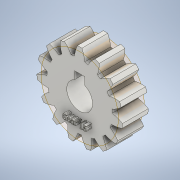
# Autodesk Inventor part: Spur Gear15
Saved by Autodesk Inventor 2021 (Build 250183000, 183)
## iProperties
CustomPartVersion: 1
Created: 2021-04-10
Part Number: Spur Gear15
Material: Steel
Document SubType Name: Modeling
Designer: Nabeel Azafer
Categories: <?xml version="1.0" encoding="UTF-16"?> <MemberInstance><Categories><FamilyTemplate><FamilyTemplateParameter ValueType="xs:double" Id="1" ObjectReferenceKey="da_z" ObjectType="kUserParameterObject"/><FamilyTemplateParameter ValueType="xs:double" Id="2" ObjectReferenceKey="da_b" ObjectType="kUserParameterObject"/><FamilyTemplateParameter ValueType="xs:double" Id="3" ObjectReferenceKey="da_beta" ObjectType="kUserParameterObject"/><FamilyTemplateParameter ValueType="xs:double" Id="4" ObjectReferenceKey="da_da" ObjectType="kUserParameterObject"/><FamilyTemplateParameter ValueType="xs:double" Id="5" ObjectReferenceKey="da_aw" ObjectType="kUserParameterObject"/><FamilyTemplateParameter ValueType="xs:string" Id="6" ObjectReferenceKey="EAIAABAAAACIAQAAAAAAAIAAAAAAAAAA" ObjectType="83910656" SubObjectId="SurfaceGeometry"/></FamilyTemplate><ParamToTemplateMap><ParamToTemplate CategoryParameter="//CategoryParameter[@InternalName='046C89C9-8512-4d59-83FE-43B91F4F132A']" TemplateParameter="1"/><ParamToTemplate CategoryParameter="//CategoryParameter[@InternalName='2552DF32-E462-4b46-AEBF-C6C7768E72AC']" TemplateParameter="2"/><ParamToTemplate CategoryParameter="//CategoryParameter[@InternalName='C9EE641D-15FC-4fae-A226-E94C4372FDD7']" TemplateParameter="3"/><ParamToTemplate><ParamToTemplate CategoryParameter="//CategoryParameter[@InternalName='00B6519A-459B-49c7-AD84-2E56D39A5744']" ConstantValue="0.000000"/></ParamToTemplate><ParamToTemplate><ParamToTemplate CategoryParameter="//CategoryParameter[@InternalName='04B31F0E-C7A6-4894-AA32-9629BEFACF47']" ConstantValue="0.800000"/></ParamToTemplate><ParamToTemplate><ParamToTemplate CategoryParameter="//CategoryParameter[@InternalName='43CBEC2E-7847-49e7-A936-2F7889FCB2D9']" ConstantValue="0.350000"/></ParamToTemplate><ParamToTemplate><ParamToTemplate CategoryParameter="//CategoryParameter[@InternalName='B1EFC894-105D-4ebd-86BF-FA20ED196853']" ConstantValue="0.500000"/></ParamToTemplate><ParamToTemplate><ParamToTemplate CategoryParameter="//CategoryParameter[@InternalName='51175063-3D10-4879-93E8-6246FE8B403D']" ConstantValue="2060000000.000000"/></ParamToTemplate><ParamToTemplate><ParamToTemplate CategoryParameter="//CategoryParameter[@InternalName='A3A52E27-4454-46a9-B0BD-C932399B70AF']" ConstantValue="0.300000"/></ParamToTemplate><ParamToTemplate><ParamToTemplate CategoryParameter="//CategoryParameter[@InternalName='91B76062-C214-41d9-B1B9-14D2AB99603D']" ConstantValue="0.100000"/></ParamToTemplate><ParamToTemplate><ParamToTemplate CategoryParameter="//CategoryParameter[@InternalName='374E806E-8B8A-4dda-A9AA-1039D6500AD2']" ConstantValue="10.000000"/></ParamToTemplate><ParamToTemplate><ParamToTemplate CategoryParameter="//CategoryParameter[@InternalName='2D373A89-B862-43d6-8D0B-0CBF12AB9F6C']" ConstantValue="0.349066"/></ParamToTemplate><ParamToTemplate CategoryParameter="//CategoryParameter[@InternalName='37777632-D6A2-4fac-9D53-DB8ACD95C989']" TemplateParameter="4"/><ParamToTemplate CategoryParameter="//CategoryParameter[@InternalName='FD1017F1-B727-4f7e-9707-0F86F1FF9423']" TemplateParameter="5"/><ParamToTemplate><ParamToTemplate CategoryParameter="//CategoryParameter[@InternalName='9E1B4470-B2D3-4ff1-B813-535BB4CDF51A']" ConstantValue="3520000.000000"/></ParamToTemplate><ParamToTemplate><ParamToTemplate CategoryParameter="//CategoryParameter[@InternalName='F8452263-BFF6-458c-9FB1-07C4B99E95CD']" ConstantValue="11400000.000000"/></ParamToTemplate><ParamToTemplate><ParamToTemplate CategoryParameter="//CategoryParameter[@InternalName='3E3BB259-FD49-497f-8171-6EBC954A3479']" ConstantValue="2.000000"/></ParamToTemplate><ParamToTemplate CategoryParameter="//CategoryParameter[@InternalName='27C3BAF2-7550-4e4b-AE2C-0DB134B7D9B7']" TemplateParameter="6"/></ParamToTemplateMap><Category DisplayName="Gear" InternalName="DC85795E-93AB-48d5-8EEE-5A27447B64BD" Mnemonic="Gear"><CategoryParameter DisplayName="z" InternalName="046C89C9-8512-4d59-83FE-43B91F4F132A" Mnemonic="z"/><CategoryParameter DisplayName="b" InternalName="2552DF32-E462-4b46-AEBF-C6C7768E72AC" Mnemonic="b"/><CategoryParameter DisplayName="||b|" InternalName="C9EE641D-15FC-4fae-A226-E94C4372FDD7" Mnemonic="beta"/><CategoryParameter DisplayName="x" InternalName="00B6519A-459B-49c7-AD84-2E56D39A5744" Mnemonic="x"/><CategoryParameter DisplayName="a*" InternalName="04B31F0E-C7A6-4894-AA32-9629BEFACF47" Mnemonic="a"/><CategoryParameter DisplayName="c*" InternalName="43CBEC2E-7847-49e7-A936-2F7889FCB2D9" Mnemonic="c"/><CategoryParameter DisplayName="r|.f|*" InternalName="B1EFC894-105D-4ebd-86BF-FA20ED196853" Mnemonic="rf"/><CategoryParameter DisplayName="E" InternalName="51175063-3D10-4879-93E8-6246FE8B403D" Mnemonic="E"/><CategoryParameter DisplayName="||m|" InternalName="A3A52E27-4454-46a9-B0BD-C932399B70AF" Mnemonic="mi"/><Category DisplayName="SpurGear" InternalName="26C5A22E-A91E-4dfd-A3B3-23CCAFAE1764" Mnemonic="SpurGear"><CategoryParameter DisplayName="m" InternalName="91B76062-C214-41d9-B1B9-14D2AB99603D" Mnemonic="m"/><CategoryParameter DisplayName="P" InternalName="374E806E-8B8A-4dda-A9AA-1039D6500AD2" Mnemonic="PP"/><CategoryParameter DisplayName="||a|" InternalName="2D373A89-B862-43d6-8D0B-0CBF12AB9F6C" Mnemonic="alpha"/><CategoryParameter DisplayName="d|.a|" InternalName="37777632-D6A2-4fac-9D53-DB8ACD95C989" Mnemonic="da"/><CategoryParameter DisplayName="a|.w|" InternalName="FD1017F1-B727-4f7e-9707-0F86F1FF9423" Mnemonic="aw"/><CategoryParameter DisplayName="||s||.Flim|" InternalName="9E1B4470-B2D3-4ff1-B813-535BB4CDF51A" Mnemonic="sFlim"/><CategoryParameter DisplayName="||s||.Hlim|" InternalName="F8452263-BFF6-458c-9FB1-07C4B99E95CD" Mnemonic="sHlim"/><CategoryParameter DisplayName="type" InternalName="3E3BB259-FD49-497f-8171-6EBC954A3479" Mnemonic="type"/><CategoryParameter DisplayName="PitchDiameter" InternalName="27C3BAF2-7550-4e4b-AE2C-0DB134B7D9B7" Mnemonic="IDS_PITCHDIAM"/></Category></Category></Categories></MemberInstance>
Density: 7.85 g/cm^3
Appearance: Steel
Mass: 10.3734 g
Surface Area: 10.947 cm^2
Volume: 1.32145 cm^3
Author: Nabeel Azafer
Autodesk Inventor part; units mm, degrees
ref_plane "YZ Plane" through (0, 0, 0) normal (1, 0, 0) x (0, 1, 0)
ref_plane "XZ Plane" through (0, 0, 0) normal (0, 1, 0) x (-1, 0, 0)
ref_plane "XY Plane" through (0, 0, 0) normal (0, 0, 1) x (1, 0, 0)
sketch "Sketch1" plane through (0, 0, 0) normal (0, 0, 1) x (1, 0, 0)
  circle A0 centre (0, 0) radius 8.3
  dimension "d0" = 16.6
  constraints: 1 centre point
  measures "d0" diameter of A0
extrude "Extrusion1" add sketch "Sketch1" along normal blind 5
ref_plane "Work Plane2" through (0, 0, 2.5) normal (0, 0, 1) x (1, 0, 0)
sketch "Sketch2" plane through (0, 0, 0) normal (0, 0, -1) x (-1, 0, 0)
  circle A0 centre (0, 0) radius 8.3 projected
  circle A1 centre (0, 0) radius 7.5
  dimension "d3" = 15
  constraints: 1 centre point, 1 coincident
  measures "d3" diameter of A1
surface extrude "Pitch Diameter" sketch "Sketch2" against normal through all shown yes curves A1
ref_plane "Work Plane8" through (0, 0, 0) normal (0.9781476, 0.2079117, 0) x (0, 0, 1)
ref_plane "Work Plane9" through (0, 0, 0) normal (1, 0, 0) x (0, 1, 0)
spur gear teeth "Spur Gear" teeth 15 pitch diameter 15 tip diameter 16.6 root diameter 12.7 face width 8 start plane through (0, 0, 0) normal (0, 0, -1) x (-1, 0, 0)
sketch "Sketch4" plane through (0, 0, 5) normal (0, 0, 1) x (1, 0, 0)
  circle A0 centre (0, 0) radius 2.5
  line L0 (-1, 2.2913) -> (1, 2.2913)
  line L1 (1, 2.2913) -> (1, 3.7913)
  line L2 (1, 3.7913) -> (-1, 3.7913)
  line L3 (-1, 3.7913) -> (-1, 2.2913)
  dimension "d57" = 5
  dimension "d58" = 2
  dimension "d59" = 1.5
  constraints: 8 end point, 2 parallel, 1 coincident, 1 horizontal, 1 perpendicular, 3 other
  measures "d58" distance of L2.end L1.end
  measures "d59" distance of L1.end L0.end
extrude "Extrusion2" cut sketch "Sketch4" against normal blind 5
sketch "Sketch5" plane through (0, 0, 5) normal (0, 0, 1) x (1, 0, 0)
  line L0 (-2.4127, -3.3956) -> (4.2445, -3.3956) construction
  line L1 (4.2445, -3.3956) -> (4.2445, -5.5849) construction
  line L2 (4.2445, -5.5849) -> (-2.4127, -5.5849) construction
  line L3 (-2.4127, -5.5849) -> (-2.4127, -3.3956) construction
  spline S0 degree 2 poles (-1.8924, -4.4329) (-1.9986, -4.4329) (-2.1744, -4.3681) (-2.2376, -4.3024) knots 0 0 0 1 2 2 2
  spline S1 degree 2 poles (-2.2376, -4.3024) (-2.3008, -4.236) (-2.3681, -4.0399) (-2.3681, -3.9126) knots 0 0 0 1 2 2 2
  spline S2 degree 2 poles (-2.3681, -3.9126) (-2.3681, -3.7919) (-2.3, -3.6006) (-2.2368, -3.5326) knots 0 0 0 1 2 2 2
  spline S3 degree 2 poles (-2.2368, -3.5326) (-2.176, -3.4669) (-1.9978, -3.3956) (-1.8916, -3.3956) knots 0 0 0 1 2 2 2
  spline S4 degree 2 poles (-1.8916, -3.3956) (-1.8405, -3.3956) (-1.7482, -3.4102) (-1.706, -3.4232) knots 0 0 0 1 2 2 2
  spline S5 degree 2 poles (-1.706, -3.4232) (-1.672, -3.4329) (-1.5893, -3.4685) (-1.5642, -3.4815) knots 0 0 0 1 2 2 2
  line L4 (-1.5642, -3.4815) -> (-1.5642, -3.642)
  line L5 (-1.5642, -3.642) -> (-1.5756, -3.642)
  spline S6 degree 2 poles (-1.5756, -3.642) (-1.6007, -3.6201) (-1.6534, -3.5804) (-1.702, -3.5577) knots 0 0 0 1 2 2 2
  spline S7 degree 2 poles (-1.702, -3.5577) (-1.7425, -3.5374) (-1.847, -3.5107) (-1.907, -3.5107) knots 0 0 0 1 2 2 2
  spline S8 degree 2 poles (-1.907, -3.5107) (-2.0512, -3.5107) (-2.2295, -3.7279) (-2.2295, -3.9086) knots 0 0 0 1 2 2 2
  spline S9 degree 2 poles (-2.2295, -3.9086) (-2.2295, -4.0091) (-2.1825, -4.1598) (-2.138, -4.2117) knots 0 0 0 1 2 2 2
  spline S10 degree 2 poles (-2.138, -4.2117) (-2.095, -4.2635) (-1.9735, -4.3178) (-1.8973, -4.3178) knots 0 0 0 1 2 2 2
  spline S11 degree 2 poles (-1.8973, -4.3178) (-1.8414, -4.3178) (-1.7295, -4.3016) (-1.6914, -4.2854) knots 0 0 0 1 2 2 2
  line L6 (-1.6914, -4.2854) -> (-1.6914, -4.0269)
  line L7 (-1.6914, -4.0269) -> (-1.9232, -4.0269)
  line L8 (-1.9232, -4.0269) -> (-1.9232, -3.9102)
  line L9 (-1.9232, -3.9102) -> (-1.5602, -3.9102)
  line L10 (-1.5602, -3.9102) -> (-1.5602, -4.347)
  spline S12 degree 2 poles (-1.5602, -4.347) (-1.5853, -4.3583) (-1.6712, -4.3932) (-1.7076, -4.4037) knots 0 0 0 1 2 2 2
  spline S13 degree 2 poles (-1.7076, -4.4037) (-1.7571, -4.4183) (-1.8365, -4.4329) (-1.8924, -4.4329) knots 0 0 0 1 2 2 2
  spline S14 degree 2 poles (-1.0772, -4.4305) (-1.2571, -4.4305) (-1.4548, -4.2287) (-1.4548, -4.0423) knots 0 0 0 1 2 2 2
  spline S15 degree 2 poles (-1.4548, -4.0423) (-1.4548, -3.8591) (-1.2628, -3.642) (-1.108, -3.642) knots 0 0 0 1 2 2 2
  spline S16 degree 2 poles (-1.108, -3.642) (-1.0383, -3.642) (-0.9305, -3.6825) (-0.8908, -3.7254) knots 0 0 0 1 2 2 2
  spline S17 degree 2 poles (-0.8908, -3.7254) (-0.8503, -3.7684) (-0.8073, -3.8924) (-0.8073, -3.9823) knots 0 0 0 1 2 2 2
  line L11 (-0.8073, -3.9823) -> (-0.8073, -4.0512)
  line L12 (-0.8073, -4.0512) -> (-1.3268, -4.0512)
  spline S18 degree 2 poles (-1.3268, -4.0512) (-1.3268, -4.1817) (-1.1955, -4.3202) (-1.0788, -4.3202) knots 0 0 0 1 2 2 2
  spline S19 degree 2 poles (-1.0788, -4.3202) (-1.0375, -4.3202) (-0.9572, -4.3016) (-0.9248, -4.287) knots 0 0 0 1 2 2 2
  spline S20 degree 2 poles (-0.9248, -4.287) (-0.8908, -4.2708) (-0.8438, -4.2425) (-0.8284, -4.2295) knots 0 0 0 1 2 2 2
  line L13 (-0.8284, -4.2295) -> (-0.8211, -4.2295)
  line L14 (-0.8211, -4.2295) -> (-0.8211, -4.3673)
  spline S21 degree 2 poles (-0.8211, -4.3673) (-0.843, -4.3762) (-0.9094, -4.4021) (-0.9354, -4.4094) knots 0 0 0 1 2 2 2
  spline S22 degree 2 poles (-0.9354, -4.4094) (-0.9718, -4.4199) (-1.0318, -4.4305) (-1.0772, -4.4305) knots 0 0 0 1 2 2 2
  spline S23 degree 2 poles (-0.9305, -3.9548) (-0.9321, -3.9037) (-0.9532, -3.8292) (-0.9735, -3.804) knots 0 0 0 1 2 2 2
  spline S24 degree 2 poles (-0.9735, -3.804) (-0.9953, -3.7757) (-1.0642, -3.7457) (-1.1153, -3.7457) knots 0 0 0 1 2 2 2
  spline S25 degree 2 poles (-1.1153, -3.7457) (-1.1655, -3.7457) (-1.236, -3.7757) (-1.2652, -3.8049) knots 0 0 0 1 2 2 2
  spline S26 degree 2 poles (-1.2652, -3.8049) (-1.2935, -3.8348) (-1.3227, -3.907) (-1.3268, -3.9548) knots 0 0 0 1 2 2 2
  line L15 (-1.3268, -3.9548) -> (-0.9305, -3.9548)
  spline S27 degree 2 poles (-0.2611, -4.334) (-0.2765, -4.3454) (-0.3284, -4.3859) (-0.3527, -4.398) knots 0 0 0 1 2 2 2
  spline S28 degree 2 poles (-0.3527, -4.398) (-0.3859, -4.4159) (-0.4483, -4.4345) (-0.5051, -4.4345) knots 0 0 0 1 2 2 2
  spline S29 degree 2 poles (-0.5051, -4.4345) (-0.5512, -4.4345) (-0.6347, -4.3997) (-0.6663, -4.3681) knots 0 0 0 1 2 2 2
  spline S30 degree 2 poles (-0.6663, -4.3681) (-0.6963, -4.3373) (-0.7328, -4.2465) (-0.7328, -4.1963) knots 0 0 0 1 2 2 2
  spline S31 degree 2 poles (-0.7328, -4.1963) (-0.7328, -4.1185) (-0.6671, -4.0083) (-0.5958, -3.9767) knots 0 0 0 1 2 2 2
  spline S32 degree 2 poles (-0.5958, -3.9767) (-0.5326, -3.9475) (-0.3608, -3.9256) (-0.2611, -3.9199) knots 0 0 0 1 2 2 2
  line L16 (-0.2611, -3.9199) -> (-0.2611, -3.8956)
  spline S33 degree 2 poles (-0.2611, -3.8956) (-0.2611, -3.8519) (-0.2879, -3.7976) (-0.3122, -3.7822) knots 0 0 0 1 2 2 2
  spline S34 degree 2 poles (-0.3122, -3.7822) (-0.3365, -3.7668) (-0.4062, -3.757) (-0.4435, -3.757) knots 0 0 0 1 2 2 2
  spline S35 degree 2 poles (-0.4435, -3.757) (-0.4872, -3.757) (-0.6055, -3.783) (-0.6647, -3.8081) knots 0 0 0 1 2 2 2
  line L17 (-0.6647, -3.8081) -> (-0.672, -3.8081)
  line L18 (-0.672, -3.8081) -> (-0.672, -3.6792)
  spline S36 degree 2 poles (-0.672, -3.6792) (-0.6371, -3.6695) (-0.5067, -3.6452) (-0.4427, -3.6452) knots 0 0 0 1 2 2 2
  spline S37 degree 2 poles (-0.4427, -3.6452) (-0.3649, -3.6452) (-0.2587, -3.6695) (-0.2166, -3.7011) knots 0 0 0 1 2 2 2
  spline S38 degree 2 poles (-0.2166, -3.7011) (-0.1752, -3.7319) (-0.1347, -3.83) (-0.1347, -3.9005) knots 0 0 0 1 2 2 2
  line L19 (-0.1347, -3.9005) -> (-0.1347, -4.4134)
  line L20 (-0.1347, -4.4134) -> (-0.2611, -4.4134)
  line L21 (-0.2611, -4.4134) -> (-0.2611, -4.334)
  line L22 (-0.2611, -4.2287) -> (-0.2611, -4.0204)
  spline S39 degree 2 poles (-0.2611, -4.0204) (-0.3065, -4.0245) (-0.4435, -4.0382) (-0.4864, -4.0512) knots 0 0 0 1 2 2 2
  spline S40 degree 2 poles (-0.4864, -4.0512) (-0.5367, -4.0666) (-0.6023, -4.1306) (-0.6023, -4.1873) knots 0 0 0 1 2 2 2
  spline S41 degree 2 poles (-0.6023, -4.1873) (-0.6023, -4.2522) (-0.5294, -4.3178) (-0.4597, -4.3178) knots 0 0 0 1 2 2 2
  spline S42 degree 2 poles (-0.4597, -4.3178) (-0.4005, -4.3178) (-0.3033, -4.2668) (-0.2611, -4.2287) knots 0 0 0 1 2 2 2
  line L23 (0.4406, -3.7984) -> (0.4342, -3.7984)
  spline S43 degree 2 poles (0.4342, -3.7984) (0.4196, -3.7943) (0.388, -3.7927) (0.3661, -3.7927) knots 0 0 0 1 2 2 2
  spline S44 degree 2 poles (0.3661, -3.7927) (0.315, -3.7927) (0.2146, -3.8373) (0.1692, -3.881) knots 0 0 0 1 2 2 2
  line L24 (0.1692, -3.881) -> (0.1692, -4.4134)
  line L25 (0.1692, -4.4134) -> (0.0428, -4.4134)
  line L26 (0.0428, -4.4134) -> (0.0428, -3.663)
  line L27 (0.0428, -3.663) -> (0.1692, -3.663)
  line L28 (0.1692, -3.663) -> (0.1692, -3.7749)
  spline S45 degree 2 poles (0.1692, -3.7749) (0.2381, -3.7133) (0.341, -3.663) (0.3896, -3.663) knots 0 0 0 1 2 2 2
  spline S46 degree 2 poles (0.3896, -3.663) (0.409, -3.663) (0.4285, -3.6647) (0.4406, -3.6671) knots 0 0 0 1 2 2 2
  line L29 (0.4406, -3.6671) -> (0.4406, -3.7984)
  line L30 (1.516, -4.4134) -> (1.0282, -4.4134)
  line L31 (1.0282, -4.4134) -> (1.0282, -4.3113)
  line L32 (1.0282, -4.3113) -> (1.2097, -4.3113)
  line L33 (1.2097, -4.3113) -> (1.2097, -3.6412)
  line L34 (1.2097, -3.6412) -> (1.0282, -3.6412)
  line L35 (1.0282, -3.6412) -> (1.0282, -3.5496)
  spline S47 degree 2 poles (1.0282, -3.5496) (1.1311, -3.5496) (1.2283, -3.4912) (1.2348, -3.4102) knots 0 0 0 1 2 2 2
  line L36 (1.2348, -3.4102) -> (1.3385, -3.4102)
  line L37 (1.3385, -3.4102) -> (1.3385, -4.3113)
  line L38 (1.3385, -4.3113) -> (1.516, -4.3113)
  line L39 (1.516, -4.3113) -> (1.516, -4.4134)
  spline S48 degree 2 poles (2.3061, -4.0958) (2.3061, -4.1679) (2.2599, -4.2911) (2.2178, -4.3365) knots 0 0 0 1 2 2 2
  spline S49 degree 2 poles (2.2178, -4.3365) (2.1757, -4.3818) (2.0501, -4.4345) (1.9723, -4.4345) knots 0 0 0 1 2 2 2
  spline S50 degree 2 poles (1.9723, -4.4345) (1.9009, -4.4345) (1.7616, -4.4029) (1.7105, -4.3778) knots 0 0 0 1 2 2 2
  line L40 (1.7105, -4.3778) -> (1.7105, -4.236)
  line L41 (1.7105, -4.236) -> (1.7202, -4.236)
  spline S51 degree 2 poles (1.7202, -4.236) (1.7356, -4.2473) (1.7932, -4.2765) (1.828, -4.2895) knots 0 0 0 1 2 2 2
  spline S52 degree 2 poles (1.828, -4.2895) (1.8677, -4.3032) (1.9334, -4.3186) (1.9747, -4.3186) knots 0 0 0 1 2 2 2
  spline S53 degree 2 poles (1.9747, -4.3186) (2.0152, -4.3186) (2.0914, -4.2895) (2.1189, -4.2579) knots 0 0 0 1 2 2 2
  spline S54 degree 2 poles (2.1189, -4.2579) (2.1441, -4.2279) (2.17, -4.1484) (2.17, -4.095) knots 0 0 0 1 2 2 2
  spline S55 degree 2 poles (2.17, -4.095) (2.17, -4.0415) (2.1408, -3.9734) (2.1133, -3.9507) knots 0 0 0 1 2 2 2
  spline S56 degree 2 poles (2.1133, -3.9507) (2.0849, -3.9256) (2.0006, -3.9045) (1.9496, -3.9045) knots 0 0 0 1 2 2 2
  spline S57 degree 2 poles (1.9496, -3.9045) (1.8945, -3.9045) (1.7851, -3.9215) (1.7518, -3.9288) knots 0 0 0 1 2 2 2
  line L42 (1.7518, -3.9288) -> (1.7518, -3.4134)
  line L43 (1.7518, -3.4134) -> (2.3005, -3.4134)
  line L44 (2.3005, -3.4134) -> (2.3005, -3.5309)
  line L45 (2.3005, -3.5309) -> (1.8807, -3.5309)
  line L46 (1.8807, -3.5309) -> (1.8807, -3.7976)
  spline S58 degree 2 poles (1.8807, -3.7976) (1.905, -3.7943) (1.952, -3.7919) (1.9714, -3.7919) knots 0 0 0 1 2 2 2
  spline S59 degree 2 poles (1.9714, -3.7919) (2.0484, -3.7919) (2.1546, -3.817) (2.2032, -3.8543) knots 0 0 0 1 2 2 2
  spline S60 degree 2 poles (2.2032, -3.8543) (2.2526, -3.8916) (2.3061, -4.005) (2.3061, -4.0958) knots 0 0 0 1 2 2 2
  point P0 (0, 0)
  constraints: 2 other
emboss "Emboss1" sketch "Sketch5" operation add depth 1 direction (0, 0, -1)
equation "\"d0\" = da_da"
equation "\"d3\" = da_d"
equation "\"d60\" = d57"
equation "\"d16\" = da_aw"
equation "\"d43\" = da_aw"
equation "\"d46\" = da_aw"
equation "\"da_da\" = 16.6"
equation "\"da_d\" = 15"
equation "\"da_aw\" = 22.5"
body "Solid1"
body "Srf1"
